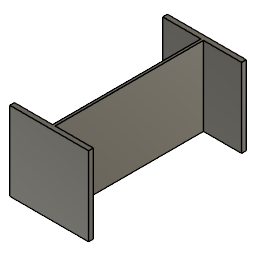
軽H-200×100×3.2×6.0 (Autodesk Fusion 360 design; units mm, degrees)
Autodesk Fusion 360 part; units mm, degrees
sketch "スケッチ1" plane through (0, 0, 0) normal (0, 0, 1) x (1, 0, 0)
  line L0 (0, -100) -> (0, 100)
  line L1 (-50, 100) -> (50, 100)
  line L2 (-50, -100) -> (50, -100)
  line L3 (-50, 94) -> (50, 94)
  line L4 (-50, -94) -> (50, -94)
  line L5 (1.6, -100) -> (1.6, 100)
  line L6 (-1.6, -100) -> (-1.6, 100)
  line L7 (50, 100) -> (50, 94)
  line L8 (-50, 100) -> (-50, 94)
  line L9 (50, -94) -> (50, -100)
  line L10 (-50, -94) -> (-50, -100)
  dimension "d1" = 200
  dimension "d2" = 100
  dimension "d3" = 100
  dimension "d4" = 6
  dimension "d5" = -6
  dimension "d6" = 1.6
  dimension "d7" = -1.6
  constraint vertical L0
  constraint midpoint origin L0
  constraint perpendicular L0 L1
  constraint midpoint L0.end L1
  constraint horizontal L2
  constraint midpoint L0.start L2
  constraint perpendicular L3 L7
  constraint perpendicular L3 L8
  constraint perpendicular L2 L9
  constraint perpendicular L2 L10
  measures "d1" distance of L0.start L0.end
  measures "d2" distance of L1.start L1.end
  measures "d3" distance of L2.start L2.end
extrude "押し出し1" add sketch "スケッチ1" along normal blind 100
